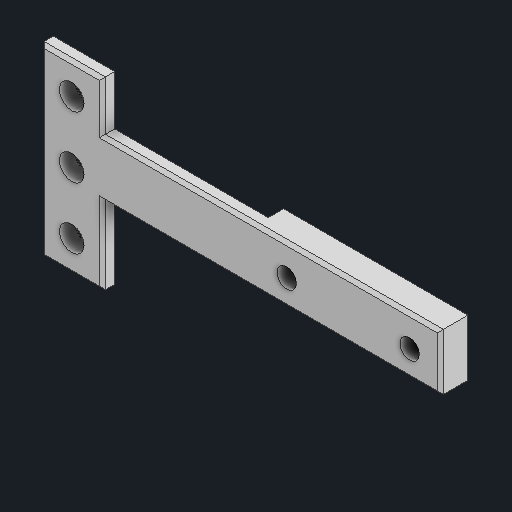
# Autodesk Inventor part: Falcon T
Saved by Autodesk Inventor 2023 (Build 270158000, 158)
## iProperties
Created: 2022-05-02
Part Number: Falcon T
Material: Generic
Document SubType Name: Modeling
Designer: FizzyApple12
Density: 1 g/cm^3
Appearance: Default
Author: FizzyApple12
Autodesk Inventor part; units mm, degrees
ref_plane "YZ Plane" through (0, 0, 0) normal (1, 0, 0) x (0, 1, 0)
ref_plane "XZ Plane" through (0, 0, 0) normal (0, 1, 0) x (-1, 0, 0)
sketch "Sketch1" plane through (0, 0, 0) normal (0, 0, 1) x (1, 0, 0)
  circle A0 centre (6.35, 19.05) radius 1.9812 projected
  circle A1 centre (6.35, 31.75) radius 1.9812 projected
  circle A2 centre (6.35, 44.45) radius 1.9812 projected
  line L0 (0, 12.7) -> (12.7, 12.7)
  line L1 (12.7, 12.7) -> (12.7, 50.8)
  line L2 (12.7, 50.8) -> (0, 50.8)
  line L3 (0, 50.8) -> (0, 12.7)
  circle A3 centre (76.2, 34.175) radius 2.0193 projected
  circle A4 centre (50.8, 34.175) radius 2.0193 projected
  line L4 (82.55, 40.525) -> (12.7, 40.525)
  line L5 (12.7, 40.525) -> (12.7, 28.875)
  line L6 (12.7, 28.875) -> (82.55, 28.875)
  line L7 (82.55, 28.875) -> (82.55, 40.525)
  line L8 (80.475, 28.875) -> (71.925, 28.875) projected
  point P0 (0, 0)
  point P1 (12.7, 40.525)
  dimension "d0" = 6.35
  dimension "d1" = 6.35
  dimension "d2" = 6.35
  dimension "d3" = 6.35
  dimension "d4" = 6.35
  dimension "d5" = 6.35
  constraints: 16 end point, 4 parallel, 2 horizontal, 2 perpendicular, 2 point on line
  measures "d0" distance from line of L0 A0.centre
  measures "d1" distance from line of L3 A0.centre
  measures "d2" distance from line of A0.centre L1
  measures "d3" distance from line of A2.centre L2
  measures "d4" distance from line of L7 A3.centre
  measures "d5" distance from line of L4 A3.centre
extrude "Extrusion1" add sketch "Sketch1" along normal blind 3.175
sketch "Sketch2" plane through (0, 0, 3.175) normal (0, 0, 1) x (1, 0, 0)
  circle A0 centre (6.35, 44.45) radius 1.9812 projected
  circle A1 centre (6.35, 31.75) radius 1.9812 projected
  circle A2 centre (6.35, 19.05) radius 1.9812 projected
  point P0 (0, 0)
  constraints: 3 coincident
hole "Hole1" at (6.35, 44.45, 3.175) at (6.35, 31.75, 3.175) at (6.35, 19.05, 3.175) direction (0, 0, -1) diameter 5.1054 depth 13.6144 clearance for "Flat Head Machine Screw (82)" size "#10" standard "Ansi Unified Screw Threads"
sketch "Sketch3" plane through (0, 0, 0) normal (0, 0, -1) x (-1, 0, 0)
  line L0 (-12.7, 28.875) -> (-82.55, 28.875) projected
  line L1 (-82.55, 40.525) -> (-12.7, 40.525) projected
  line L2 (-82.55, 28.875) -> (-44.45, 28.875)
  line L3 (-44.45, 28.875) -> (-44.45, 40.525)
  line L4 (-44.45, 40.525) -> (-82.55, 40.525)
  line L5 (-82.55, 40.525) -> (-82.55, 28.875)
  circle A0 centre (-50.8, 34.175) radius 2.0193 projected
  circle A1 centre (-76.2, 34.175) radius 2.0193 projected
  point P0 (0, 0)
  dimension "d15" = 6.35
  constraints: 8 end point, 2 parallel, 1 horizontal, 1 perpendicular, 1 point on line
  measures "d15" distance from line of L3 A0.centre
ref_plane "Work Plane1" through (71.925, 28.875, -3.175) normal (0, 0, 1) x (1, 0, 0)
extrude "Extrusion2" add sketch "Sketch3" along normal up to surface (3.175 mm away)
chamfer "Chamfer1" distance 0.635 angle 45 19 edges at (47.625, 40.525, 3.175) (12.7, 45.6625, 3.175) (6.35, 50.8, 3.175) (0, 31.75, 3.175) (6.35, 12.7, 3.175) (12.7, 20.7875, 3.175) (47.625, 28.875, 3.175) (82.55, 34.7, 3.175) (82.55, 34.7, -3.175) (63.5, 40.525, -3.175) (44.45, 34.7, -3.175) (63.5, 28.875, -3.175) (12.7, 20.7875, 0) (0, 31.75, 0) (6.35, 50.8, 0) (12.7, 45.6625, 0) (6.35, 12.7, 0) (28.575, 40.525, 0) (28.575, 28.875, 0)
body "Solid1"
